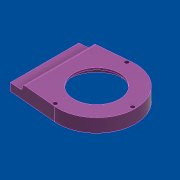
# Autodesk Inventor part: J1-sketch
Saved by Autodesk Inventor 2018 (Build 220112000, 112)
## iProperties
Created: 2019-11-26
Part Number: J1-sketch
Material: Generic
Document SubType Name: Modeling
Designer: Bunny320
Density: 1 g/cm^3
Appearance: Smooth - Purple
Author: Bunny320
## iProperties of the stored document 103-top-output_3DPrint.ipt
Created: 2019-11-29
Part Number: 103-top-output_3DPrint
Material: Generic
Document SubType Name: Modeling
Designer: mo
Density: 1 g/cm^3
Appearance: Default
Author: mo
Autodesk Inventor part; units mm, degrees
ref_plane "YZ Plane" through (0, 0, 0) normal (1, 0, 0) x (0, 1, 0)
ref_plane "XZ Plane" through (0, 0, 0) normal (0, 1, 0) x (-1, 0, 0)
ref_plane "XY Plane" through (0, 0, 0) normal (0, 0, 1) x (1, 0, 0)
sketch "Sketch1" plane through (0, 0, 0) normal (0, 0, 1) x (1, 0, 0)
  circle A0 centre (0, 0) radius 48
  circle A1 centre (141.8, 0) radius 60.5
  line L0 (136.466784, 60.264474) -> (-4.231312, 47.813136)
  line L1 (-4.231312, -47.813136) -> (136.466784, -60.264474)
  line L2 (80.8, 55.338139) -> (80.8, -55.338139)
  dimension "d0" = 96
  dimension "d1" = 121
  dimension "d2" = 141.8
  dimension "d3" = 61
  constraints: 6 end point, 4 point on circle, 4 tangent, 2 centre point, 2 point on line, 1 coincident, 1 horizontal alignment, 1 vertical
  measures "d0" diameter of A0
  measures "d1" diameter of A1
  measures "d2" distance of A1.centre point (0, 0)
  measures "d3" distance from line of A1.centre L2
extrude "Extrusion1" add sketch "Sketch1" against normal blind 21 contours L0 A1 L1 L2 | A1
sketch "Sketch2" plane through (0, 0, -21) normal (0, 0, -1) x (-1, 0, 0)
  line L0 (-80.8, -55.338139) -> (-60.3, -53.523954)
  line L1 (-60.3, -53.523954) -> (-60.3, 53.523954)
  line L2 (-60.3, 53.523954) -> (-80.8, 55.338139)
  line L3 (-80.8, 55.338139) -> (-80.8, -55.338139)
  line L4 (-136.466784, -60.264474) -> (-80.8, -55.338139)
  line L5 (-80.8, 55.338139) -> (-136.466784, 60.264474)
  line L6 (-80.8, -55.338139) -> (-80.8, 55.338139)
  point P0 (0, 0)
  dimension "d7" = 20.5
  constraints: 8 end point, 3 collinear, 1 parallel, 1 vertical
  measures "d7" distance between parallel lines of L6 L1
extrude "Extrusion2" add sketch "Sketch2" against normal blind 12
shell "Shell1" thickness 4 removed faces 1 at (111.077856, 17.841318, -21)
sketch "Sketch3" plane through (141.8, 0, -4) normal (0, 0, -1) x (-1, 0, 0)
  circle A0 centre (0, 0) radius 42
  point P0 (141.8, 0)
  dimension "d10" = 84
  constraints: 1 centre point
  measures "d10" diameter of A0
extrude "Extrusion3" cut sketch "Sketch3" against normal blind 1
sketch "Sketch4" plane through (0, 0, 0) normal (0, 0, 1) x (1, 0, 0)
  circle A0 centre (141.8, 0) radius 42 projected
  circle A1 centre (141.8, 0) radius 35.5
  point P0 (0, 0)
  dimension "d13" = 71
  constraints: 1 centre point, 1 coincident
  measures "d13" diameter of A1
extrude "Extrusion4" cut sketch "Sketch4" against normal through all contours A1
sketch "Sketch5" plane through (141.8, 0, -4) normal (0, 0, -1) x (-1, 0, 0)
  circle A0 centre (0, 0) radius 45
  circle A1 centre (0, 0) radius 48
  point P0 (141.8, 0)
  dimension "d16" = 90
  dimension "d17" = 96
  constraints: 2 centre point, 1 coincident
  measures "d16" diameter of A0
  measures "d17" diameter of A1
extrude "Extrusion5" add sketch "Sketch5" along normal blind 9
sketch "Sketch6" plane through (84.8, -51.676494, -13) normal (0, 0, -1) x (-1, 0, 0)
  line L0 (8.632076, 0.763912) -> (62.461619, 5.527656)
  line L1 (62.461619, 5.527656) -> (62.461619, 97.825331)
  line L2 (62.461619, 97.825331) -> (8.632076, 102.589076)
  line L3 (8.632076, 102.589076) -> (8.632076, 0.763912)
  line L4 (20.5, 1.814185) -> (-52.019394, -4.603552)
  line L5 (-52.019394, 107.956539) -> (20.5, 101.538802)
  constraints: 8 end point, 2 collinear, 1 parallel, 1 vertical
extrude "Extrusion6" cut sketch "Sketch6" along normal through all
fillet "Fillet1" radius 4 3 edges at (84.8, 0, -13) (80.8, 0, -9) (80.8, 0, 0)
sketch "Sketch7" plane through (141.8, 0, -4) normal (0, 0, -1) x (-1, 0, 0)
  line L0 (-52, 4) -> (-60, 4)
  line L1 (-60, 4) -> (-60, -4)
  line L2 (-60, -4) -> (-52, -4)
  line L3 (-52, -4) -> (-52, 4)
  line L4 (-52, 4) -> (-60, -4) construction
  line L5 (-60, 4) -> (-52, -4) construction
  arc A0 (4.980606, 56.280046) -> (4.980606, -56.280046) centre (0, 0) ccw
  line L6 (4.980606, -56.280046) -> (12.949463, -55.574827)
  line L7 (12.949463, -55.574827) -> (12.596853, -51.590399)
  line L8 (12.596853, -51.590399) -> (4.627997, -52.295618)
  line L9 (4.627997, -52.295618) -> (4.980606, -56.280046)
  line L10 (4.980606, 56.280046) -> (57, 51.676494)
  line L11 (4.980606, 56.280046) -> (12.949463, 55.574827)
  line L12 (12.949463, 55.574827) -> (12.596853, 51.590399)
  line L13 (12.596853, 51.590399) -> (4.627997, 52.295618)
  line L14 (4.627997, 52.295618) -> (4.980606, 56.280046)
  point P0 (141.8, 0)
  point P1 (-56, 0)
  dimension "d24" = 4
  dimension "d25" = 4
  dimension "d26" = 8
  dimension "d27" = 8
  dimension "d28" = 8
  dimension "d29" = 56
  constraints: 28 end point, 6 parallel, 4 perpendicular, 2 midpoint, 1 horizontal, 1 horizontal alignment, 1 point on line, 1 tangent
  measures "d24" distance of L11.end L12.end
  measures "d25" distance of L6.end L7.end
  measures "d26" distance of L2.end L0.start
  measures "d27" distance of L12.end L13.end
  measures "d28" distance of L7.end L8.end
  measures "d29" distance of A0.centre point (-56, 0)
extrude "Extrusion7" add sketch "Sketch7" along normal up to surface (17 mm away)
sketch "Sketch8" plane through (0, 0, 0) normal (0, 0, -1) x (-1, 0, 0)
  line L0 (-60.3, -49.508321) -> (-128.850537, -55.574827)
  line L1 (-128.850537, 55.574827) -> (-60.3, 49.508321)
  circle A0 centre (-141.8, 0) radius 35.5
  line L2 (-128.850537, -55.574827) -> (-129.203147, -51.590399)
  line L3 (-129.203147, 51.590399) -> (-128.850537, 55.574827)
  point P0 (0, 0)
  point P1 (-197.8, 0)
  point P2 (-132.834965, -55.927437)
  point P3 (-132.834965, 55.927437)
  dimension "d32" = 56
  dimension "d33" = 4
  dimension "d34" = 4
  constraints: 2 point on line, 1 horizontal alignment
  measures "d32" distance of A0.centre point (-197.8, 0)
  measures "d33" distance from line of L2 point (-132.835, -55.927)
  measures "d34" distance from line of L3 point (-132.835, 55.927)
hole "Hole1" at (197.8, 0, 0) at (132.834965, -55.927437, 0) at (132.834965, 55.927437, 0) direction (0, 0, -1) diameter 3.4 end through all counterbore diameter 6.5 counterbore depth 17 clearance for "Socket Head Cap Screw DIN EN ISO 4762" size "M3" standard "DIN"
sketch "Sketch9" plane through (0, 0, 0) normal (0, 0, 1) x (1, 0, 0)
  circle A0 centre (125.937089, 54.374793) radius 1.7
  circle A1 centre (132.834965, -55.927437) radius 1.7
  circle A2 centre (197.8, 0) radius 1.7
  point P0 (0, 0)
  constraints: 3 coincident
equation "\"d25\" = d24"
equation "\"d27\" = d26"
equation "\"d28\" = d26"
body "Solid1"
